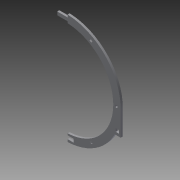
# Autodesk Inventor part: TopHoopSection_v4
Saved by Autodesk Inventor 2013 (Build 170138000, 138)
## iProperties
Created: 2013-01-17
Part Number: TopHoopSection_v4
Material: Generic
Document SubType Name: Modeling
Designer: twsass
Density: 1 g/cm^3
Author: twsass
Autodesk Inventor part; units mm, degrees
ref_plane "YZ Plane" through (0, 0, 0) normal (1, 0, 0) x (0, 1, 0)
ref_plane "XZ Plane" through (0, 0, 0) normal (0, 1, 0) x (-1, 0, 0)
ref_plane "XY Plane" through (0, 0, 0) normal (0, 0, 1) x (1, 0, 0)
sketch "Sketch1" plane through (0, 0, 0) normal (0, 0, 1) x (1, 0, 0)
  arc A0 (6.3485, -145.912) -> (6.35, 145.9119) centre (0, 0) ccw
  line L0 (6.35, -150.9919) -> (6.35, -151.13)
  line L1 (6.35, 145.9119) -> (6.35, 168.7906)
  line L2 (0, 0) -> (0, 200.5264) construction
  line L3 (6.35, 145.9119) -> (6.35, 150.9919) construction
  line L4 (6.35, 150.9919) -> (-25.4, 150.9919)
  line L5 (-25.4, 150.9919) -> (-25.4, 161.1519)
  line L6 (-25.4, 161.1519) -> (6.35, 161.1519)
  line L7 (0, -146.05) -> (0, 0) construction
  line L8 (168.91, 0) -> (168.91, -76.2)
  line L9 (168.91, -76.2) -> (150.7453, -76.2)
  line L10 (0, 0) -> (0, -63.5) construction
  line L11 (0, -63.5) -> (158.75, -63.5) construction
  line L12 (158.75, -58.7375) -> (163.83, -58.7375)
  line L13 (163.83, -58.7375) -> (163.83, -68.2625)
  line L14 (163.83, -68.2625) -> (153.67, -68.2625)
  line L15 (153.67, -68.2625) -> (153.67, -58.7375)
  line L16 (153.67, -58.7375) -> (158.75, -58.7375)
  arc A1 (6.3485, -168.7907) -> (150.7453, -76.2) centre (0, 0) ccw
  line L17 (6.35, 161.1519) -> (-6.35, 161.1519) construction
  line L18 (-6.35, 161.1519) -> (-6.35, 168.7906) construction
  line L19 (0, -146.05) -> (0, -151.13) construction
  line L20 (6.3485, -151.13) -> (25.4, -151.13)
  line L21 (25.4, -151.13) -> (25.4, -161.29)
  line L22 (25.4, -161.29) -> (6.3485, -161.29)
  arc A2 (168.91, 0) -> (6.35, 168.7906) centre (0, 0) ccw
  line L23 (0, -146.05) -> (6.3485, -145.912) construction
  line L24 (6.3485, -145.912) -> (6.3485, -151.13)
  line L25 (6.3485, -161.29) -> (6.3485, -168.7907)
  line L26 (6.3485, -145.912) -> (6.3485, -151.13) construction
  line L27 (6.3485, -161.29) -> (6.3485, -184.4747) construction
  line L28 (0, 0) -> (762, -1319.8227) construction
  line L29 (0, 0) -> (1524, 0) construction
  line L30 (0, 0) -> (158.4844, 274.503) construction
  line L31 (0, 0) -> (316.9688, 0) construction
  line L32 (76.2, -131.9823) -> (78.9496, -130.3948)
  line L33 (78.9496, -130.3948) -> (82.1246, -135.894)
  line L34 (82.1246, -135.894) -> (76.6254, -139.069)
  line L35 (76.6254, -139.069) -> (73.4504, -133.5698)
  line L36 (73.4504, -133.5698) -> (76.2, -131.9823)
  line L37 (152.4, 0) -> (152.4, -3.175)
  line L38 (152.4, -3.175) -> (158.75, -3.175)
  line L39 (158.75, -3.175) -> (158.75, 3.175)
  line L40 (158.75, 3.175) -> (152.4, 3.175)
  line L41 (152.4, 3.175) -> (152.4, -3.175)
  line L42 (73.4504, 133.5698) -> (76.6254, 139.069)
  line L43 (76.6254, 139.069) -> (82.1246, 135.894)
  line L44 (82.1246, 135.894) -> (78.9496, 130.3948)
  line L45 (78.9496, 130.3948) -> (73.4504, 133.5698)
  point P0 (6.35, -145.9119)
  point P1 (0.0447, 168.91)
  point P2 (6.3947, 145.9099)
  dimension "d51" = 292.1
  dimension "d72" = 6.35
  dimension "d73" = 5.08
  dimension "d75" = 31.75
  dimension "d76" = 10.16
  dimension "d82" = 76.2
  dimension "d86" = 63.5
  dimension "d87" = 158.75
  dimension "d89" = 4.7625
  dimension "d90" = 5.08
  dimension "d91" = 9.525
  dimension "d92" = 10.16
  dimension "d93" = 4.7625
  dimension "d100" = 12.7
  dimension "d101" = 5.08
  dimension "d103" = 25.4
  dimension "d104" = 10.16
  dimension "d105" = 6.35
  dimension "d106" = 7.5007
  dimension "d107" = 25.4
  dimension "d113" = 1524
  dimension "d114" = 60
  dimension "d115" = 60
  dimension "d121" = 3.175
  dimension "d122" = 6.35
  dimension "d123" = 152.4
  dimension "d124" = 6.35
  dimension "d125" = 3.175
  dimension "d126" = 6.35
  dimension "d127" = 6.35
  dimension "d128" = 152.4
  dimension "d130" = 6.35
  dimension "d131" = 6.35
  dimension "d132" = 6.35
  dimension "d133" = 3.175
  dimension "d134" = 152.4
  constraints: 92 end point, 22 perpendicular, 10 parallel, 8 point on circle, 8 point on line, 5 collinear, 3 centre point, 2 equal length, 2 horizontal, 1 coincident, 1 tangent, 1 vertical, 2 other
  measures "d51" diameter of A0
  measures "d72" distance between parallel lines of L1 L2
  measures "d73" distance of L1.start L3.end
  measures "d75" distance of L3.end L4.end
  measures "d76" distance of L4.end L5.end
  measures "d82" distance of L8.start L8.end
  measures "d86" distance of L2.start L10.end
  measures "d87" distance of L10.end L11.end
  measures "d89" distance of L11.end L12.start
  measures "d90" distance of L12.start L12.end
  measures "d91" distance of L12.end L13.end
  measures "d92" distance of L13.end L14.end
  measures "d93" distance between parallel lines of L11 L16
  measures "d100" distance of L6.end L17.end
  measures "d101" distance of L7.start L19.end
  measures "d103" distance of L19.end L20.end
  measures "d104" distance of L20.end L21.end
  measures "d105" distance of L23.end L7.start
  measures "d106" distance from line of L25.end L22
  measures "d107" distance from line of L7.start L21
  measures "d113" distance of L2.start L28.end
  measures "d114" angle of L28 L29
  measures "d115" angle of L31 L30
  measures "d121" distance of L32.start L32.end
  measures "d122" distance of L33.end L34.end
  measures "d123" distance from line of A0.centre L32
  measures "d124" distance between parallel lines of L32 L34
  measures "d125" distance of L37.start L37.end
  measures "d126" distance of L37.end L38.end
  measures "d127" distance of L38.end L39.end
  measures "d128" distance from line of A0.centre L37
  measures "d130" distance of L42.start L42.end
  measures "d131" distance of L42.end L43.end
  measures "d132" distance of L43.end L44.end
  measures "d133" distance between parallel lines of L30 L44
  measures "d134" distance from line of A0.centre L45
extrude "Extrusion20" add sketch "Sketch1" along normal blind 6.35
body "Solid13"
